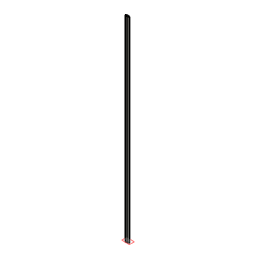
Small Strut (Autodesk Fusion 360 design; units mm, degrees)
Autodesk Fusion 360 part; units mm, degrees
sketch "Large Strut" plane through (0, 0, 0) normal (0, 0, 1) x (1, 0, 0)
  arc A0 (47.7706, 13.9652) -> (20.1744, 13.9652) centre (33.9725, -34.925) ccw
  line L0 (20.1744, 13.9652) -> (47.7706, 13.9652) construction
  line L1 (22.86, 12.8778) -> (45.085, 12.8778)
  line L2 (33.9725, 15.875) -> (33.9725, 12.8778) construction
  line L3 (22.86, 12.8778) -> (20.1744, 13.9652) construction
  line L4 (47.7706, 13.9652) -> (45.085, 12.8778) construction
  arc A1 (78.0917, 2.275) -> (47.7706, 13.9652) centre (0.204, -154.5758) ccw
  arc A2 (78.0917, -2.275) -> (78.0917, 2.275) centre (76.962, 0) ccw
  line L5 (78.0917, 2.275) -> (78.0917, -2.275) construction
  line L6 (0, 0) -> (79.502, 0) construction
  spline S0 degree 2 poles (7.4146, 7.3568) (2.7262, 4.2744) (1.778, 0) knots 0 0 0 0.96774 0.96774 0.96774 weights 1 3 1
  arc A3 (22.86, 12.8778) -> (7.4146, 7.3568) centre (44.0356, -70.728) ccw
  arc A4 (74.5112, -2.0661) -> (74.5112, 2.0661) centre (73.533, 0) ccw
  line L7 (74.5112, 2.0661) -> (74.5112, -2.0661) construction
  arc A5 (74.5112, 2.0661) -> (45.085, 12.8778) centre (-0.0506, -155.4188) ccw
  line L8 (75.819, 0) -> (79.502, 0)
  line L9 (33.9725, 12.8778) -> (33.9725, -34.925) construction
  arc A6 (20.1744, -13.9652) -> (47.7706, -13.9652) centre (33.9725, 34.925) ccw
  spline S1 degree 2 poles (7.4146, -7.3568) (2.7262, -4.2744) (1.778, 0) knots 0 0 0 0.96774 0.96774 0.96774 weights 1 3 1
  arc A7 (7.4146, -7.3568) -> (22.86, -12.8778) centre (44.0356, 70.728) ccw
  line L10 (22.86, -12.8778) -> (45.085, -12.8778)
  arc A8 (47.7706, -13.9652) -> (78.0917, -2.275) centre (0.204, 154.5758) ccw
  arc A9 (45.085, -12.8778) -> (74.5112, -2.0661) centre (-0.0506, 155.4188) ccw
  line L11 (1.778, 0) -> (0, 0)
  spline S2 degree 2 poles (0, 0) (1.0542, -5.7805) (6.2656, -9.135) knots 0 0 0 1.164804 1.164804 1.164804 weights 1 3 1
  spline S3 degree 5 poles (6.2656, -9.135) (6.8099, -9.3744) (7.8882, -9.8418) (9.4748, -10.5093) (11.5273, -11.3308) (13.9804, -12.2352) (16.3085, -13.0035) (18.4971, -13.6199) (20.5324, -14.0694) (22.4079, -14.3449) (24.1291, -14.4526) (25.3902, -14.4124) (26.2744, -14.3152) (26.8369, -14.2212) (27.1115, -14.1668) knots 0 0 0 0 0 0 0.1 0.2 0.3 0.4 0.5 0.6 0.7 0.8 0.9 1 1 1 1 1 1
  spline S4 degree 2 poles (0, 0) (1.0542, 5.7805) (6.2656, 9.135) knots 0 0 0 1.164804 1.164804 1.164804 weights 1 3 1
  spline S5 degree 5 poles (6.2656, 9.135) (6.8099, 9.3744) (7.8882, 9.8418) (9.4748, 10.5093) (11.5273, 11.3308) (13.9804, 12.2352) (16.3085, 13.0035) (18.4971, 13.6199) (20.5324, 14.0694) (22.4079, 14.3449) (24.1291, 14.4526) (25.3902, 14.4124) (26.2744, 14.3152) (26.8369, 14.2212) (27.1115, 14.1668) knots 0 0 0 0 0 0 0.1 0.2 0.3 0.4 0.5 0.6 0.7 0.8 0.9 1 1 1 1 1 1
  line L12 (3.8231, -8.0611) -> (8.7082, -10.209)
  line L13 (25.2685, -14.5318) -> (28.9545, -13.8018)
  line L14 (3.8231, 8.0611) -> (8.7082, 10.209)
  line L15 (25.2685, 14.5318) -> (28.9545, 13.8018)
  point P0 (47.7706, 13.9652)
  point P1 (20.1744, 13.9652)
  point P2 (78.0917, 2.275)
  point P3 (76.962, 0)
  point P4 (73.533, 0)
  point P5 (79.502, 0)
  point P6 (74.5112, 2.0661)
  point P7 (20.1744, 13.9652)
  point P8 (33.9725, 0)
  dimension "d6" = 22.225
  dimension "d19" = 12.8778
  dimension "d21" = 15.875
  dimension "d24" = 22.86
  dimension "d25" = 79.502
  dimension "d26" = 3.429
  dimension "d27" = 1.778
  dimension "d30" = 50.8
  dimension "d31" = 2.54
  dimension "d33" = 2.286
  dimension "d34" = 174.244
  dimension "d49" = 74.3072
  dimension "d50" = 175.1246
  constraint horizontal L0
  constraint horizontal L1
  constraint midpoint A0 L2.start
  constraint midpoint L1 L2.end
  constraint vertical L2
  constraint coincident P7 P1
  constraint coincident P0 A0.start
  constraint equal L3 L4
  constraint coincident P7 A0.end
  constraint tangent A0 A1
  constraint tangent A1 A2
  constraint coincident A1 P2
  constraint vertical L5
  constraint coincident L6.start L11.end
  constraint midpoint A2 P5
  constraint perpendicular L5 L6
  constraint coincident L6 S0.end
  constraint vertical L7
  constraint tangent A1 A5
  constraint coincident L6 P4
  constraint tangent A4 A5
  constraint symmetric L11.end L6 S2.start
  constraint symmetric A2.start L6 P2
  constraint symmetric P3 L6 A2.centre
  constraint symmetric P5 L6 L8.end
  constraint symmetric L6 A4.start P6
  constraint symmetric L6 P4 A4.centre
  constraint midpoint A4 L8.start
  constraint coincident P5 L6.end
  constraint coincident A0.centre L9.end
  constraint symmetric P0 L6 A6.end
  constraint symmetric A0 L6 A6
  constraint symmetric L1.start L6 A7.end
  constraint symmetric L1.end L6 L10.end
  constraint symmetric P7 L6 A6.start
  constraint symmetric A1 L6 A8
  constraint symmetric P2 L6 A2.start
  constraint symmetric L6 S0.start S1.start
  constraint symmetric L6 S0.end S1.end
  constraint symmetric L6 S0 S1
  constraint symmetric L6 A3 A7
  constraint symmetric L6 P6 A4.start
  constraint symmetric L6 A5 A9
  constraint midpoint S2.end L12
  constraint midpoint S3.end L13
  constraint symmetric L6 A6.start P7
  constraint symmetric L6 L11.end S2.start
  constraint symmetric L6 S2.end S4.end
  constraint symmetric L6 S2 S4
  constraint symmetric L6 S3.end S5.end
  constraint symmetric L6 L12.start L14.start
  constraint symmetric L6 L12.end L14.end
  constraint symmetric L6 L13.start L15.start
  constraint symmetric L6 L13.end L15.end
  constraint coincident L6 P8
  constraint coincident L9 P8
  measures "d6" distance of L1.start L1.end
  measures "d19" distance of L1 L6
  measures "d21" distance of L2.start L6
  measures "d24" horizontal distance of L6.start L1.start
  measures "d25" distance of L6.start P5
  measures "d26" distance of P3 P4
  measures "d27" distance of L6.start S0.end
  measures "d30" radius of A0
  measures "d31" radius of A2
  measures "d33" radius of A4
  measures "d34" radius of A5
  measures "d49" horizontal distance of A1.centre A4.start
  measures "d50" radius of A1
sketch "Small Strut" plane through (0, 0, 0) normal (0, 0, 1) x (1, 0, 0)
  line L0 (0, 0) -> (61.976, 0) construction
  line L1 (15.748, 9.7028) -> (34.798, 9.7028)
  arc A0 (36.8659, 11.3595) -> (13.6801, 11.3595) centre (25.273, -38.1) ccw
  line L2 (13.6801, 11.3595) -> (15.748, 9.7028) construction
  line L3 (36.8659, 11.3595) -> (34.798, 9.7028) construction
  arc A1 (60.8172, -1.9888) -> (60.8172, 1.9888) centre (59.69, 0) ccw
  line L4 (60.8172, 1.9888) -> (60.8172, -1.9888) construction
  line L5 (58.8343, 1.3614) -> (58.8343, -1.3614) construction
  arc A2 (60.8172, 1.9888) -> (36.8659, 11.3595) centre (16.2305, -76.6784) ccw
  arc A3 (58.8343, 1.3614) -> (34.798, 9.7028) centre (15.4476, -84.8576) ccw
  line L6 (25.273, 9.7028) -> (25.273, 12.7) construction
  spline S0 degree 2 poles (0, 0) (0.5625, 4.2011) (5.2997, 7.5955) knots 0 0 0 0.971719 0.971719 0.971719 weights 1 3 1
  spline S1 degree 2 poles (1.524, 0) (1.8308, 3.1567) (7.1158, 6.7238) knots 0 0 0 0.917957 0.917957 0.917957 weights 1 3 1
  line L7 (0, 0) -> (1.524, 0)
  line L8 (59.69, 0) -> (61.976, 0)
  arc A4 (58.8343, -1.3614) -> (58.8343, 1.3614) centre (58.1492, 0) ccw
  line L9 (59.69, 0) -> (58.1492, 0)
  arc A5 (36.8659, -11.3595) -> (60.8172, -1.9888) centre (16.2305, 76.6784) ccw
  arc A6 (34.798, -9.7028) -> (58.8343, -1.3614) centre (15.4476, 84.8576) ccw
  arc A7 (13.6801, -11.3595) -> (36.8659, -11.3595) centre (25.273, 38.1) ccw
  line L10 (15.748, -9.7028) -> (34.798, -9.7028)
  spline S2 degree 2 poles (1.524, 0) (1.8308, -3.1567) (7.1158, -6.7238) knots 0 0 0 0.917957 0.917957 0.917957 weights 1 3 1
  spline S3 degree 2 poles (0, 0) (0.5625, -4.2011) (5.2997, -7.5955) knots 0 0 0 0.971719 0.971719 0.971719 weights 1 3 1
  line L11 (13.6822, -11.36) -> (13.6769, -11.3588)
  spline S4 degree 2 poles (5.2997, 7.5955) (8.9959, 9.7972) (13.6801, 11.3595) knots 0 0 0 0.921677 0.921677 0.921677 weights 1 3 1
  spline S5 degree 2 poles (7.1158, 6.7238) (10.9615, 8.9037) (15.748, 9.7028) knots 0 0 0 0.921154 0.921154 0.921154 weights 1 3 1
  spline S6 degree 2 poles (7.1158, -6.7238) (10.9615, -8.9037) (15.748, -9.7028) knots 0 0 0 0.921154 0.921154 0.921154 weights 1 3 1
  spline S7 degree 2 poles (5.2997, -7.5955) (8.9959, -9.7972) (13.6801, -11.3595) knots 0 0 0 0.921677 0.921677 0.921677 weights 1 3 1
  line L12 (25.273, 9.7028) -> (25.273, -9.7028) construction
  point P0 (59.69, 0)
  point P1 (25.273, 0)
  dimension "d35" = 19.05
  dimension "d37" = 61.976
  dimension "d38" = 2.286
  dimension "d39" = 9.7028
  dimension "d40" = 50.8
  dimension "d41" = 12.7
  dimension "d42" = 15.748
  dimension "d43" = 1.524
  dimension "d44" = 1.524
  dimension "d45" = 90.424
  dimension "d46" = 96.52
  constraint coincident L0.start S0.start
  constraint horizontal L0
  constraint horizontal L1
  constraint equal L2 L3
  constraint perpendicular L0 L5
  constraint vertical L4
  constraint midpoint L0.end A1
  constraint coincident L0 P0
  constraint tangent A0 A2
  constraint midpoint L1 L6.start
  constraint midpoint A0 L6.end
  constraint vertical L6
  constraint tangent A1 A2
  constraint coincident L0 S1.start
  constraint coincident P0 A1.centre
  constraint coincident L0 A4.centre
  constraint tangent A3 A4
  constraint coincident A4.centre L9.end
  constraint symmetric L0 L1.start L10.start
  constraint symmetric L0 L1.end A6.start
  constraint symmetric L0 A0.end A7.start
  constraint symmetric L0 A0.start A5.start
  constraint symmetric L0 A0 A7
  constraint symmetric L0 L5.start L5.end
  constraint symmetric L0 A1.end A1.start
  constraint symmetric L0 A2 A5
  constraint symmetric L0 A3 A6
  constraint symmetric L0 S0.start L7.start
  constraint symmetric L0 S0.end S3.end
  constraint symmetric L0 S0 S3
  constraint symmetric L0 S1.start L7.end
  constraint symmetric L0 S1.end S2.end
  constraint symmetric L0 S1 S2
  constraint coincident A7 L11.start
  constraint tangent A7 L11
  constraint symmetric L0 S4 S7
  constraint symmetric L0 S5 S6
  constraint midpoint L10 L12.end
  constraint midpoint L12 P1
  measures "d35" distance of L1.start L1.end
  measures "d37" distance of L0.start L0.end
  measures "d38" radius of A1
  measures "d39" distance of L0 L1
  measures "d40" radius of A0
  measures "d41" distance of L0 L6.end
  measures "d42" horizontal distance of L0.start L1.start
  measures "d43" distance of L0.start S1.start
  measures "d44" radius of A4
  measures "d45" radius of A2
  measures "d46" radius of A3
extrude "Extrude3" add sketch "Small Strut" along normal blind 2667 contours L1 A0 A1 A2 A3 S0 S1 L7 L8 A4 L9 S4 S5 | A1 L7 L8 A4 L9 A5 A6 A7 L10 S2 S3 L11 S6 S7
equation "d19 = ( 1.014 / 2 ) * 1 in"
equation "d21 = ( 1.25 / 2 ) * 1 in"
equation "d39 = ( 0.764 / 2 ) * 1 in"
named bodies: "Small Strut"
